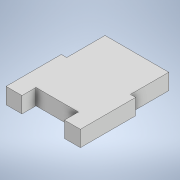
# Autodesk Inventor part: Expansiemodule
Saved by Autodesk Inventor 2021 (Build 250183000, 183)
## iProperties
Created: 2022-02-18
Part Number: Expansiemodule
Material: Generic
Document SubType Name: Modeling
Designer: woutr
Density: 1 g/cm^3
Appearance: Default
Author: woutr
Autodesk Inventor part; units mm, degrees
ref_plane "YZ Plane" through (0, 0, 0) normal (1, 0, 0) x (0, 1, 0)
ref_plane "XZ Plane" through (0, 0, 0) normal (0, 1, 0) x (-1, 0, 0)
ref_plane "XY Plane" through (0, 0, 0) normal (0, 0, 1) x (1, 0, 0)
sketch "Sketch1" plane through (0, 0, 0) normal (0, 1, 0) x (-1, 0, 0)
  line L0 (0, 0) -> (15, 0)
  line L1 (15, 0) -> (15, -13.2)
  line L2 (15, -13.2) -> (55, -13.2)
  line L3 (55, -13.2) -> (55, 0)
  line L4 (55, 0) -> (70, 0)
  line L5 (70, 0) -> (70, -52)
  line L6 (70, -52) -> (64.9, -52)
  line L7 (64.9, -52) -> (64.9, -88.1)
  line L8 (64.9, -88.1) -> (4.9, -88.1)
  line L9 (4.9, -88.1) -> (4.9, -52)
  line L10 (4.9, -52) -> (0, -52)
  line L11 (0, -52) -> (0, 0)
  dimension "d0" = 15
  dimension "d1" = 13.2
  dimension "d2" = 40
  dimension "d3" = 15
  dimension "d4" = 52
  dimension "d5" = 5.1
  dimension "d6" = 36.1
  dimension "d7" = 60
  constraints: 24 end point, 8 perpendicular, 4 point on line, 1 horizontal, 1 vertical
  measures "d0" distance of L0.start L0.end
  measures "d1" distance of L0.end L1.end
  measures "d2" distance of L1.end L2.end
  measures "d3" distance of L3.end L4.end
  measures "d4" distance of L4.end L5.end
  measures "d5" distance of L5.end L6.end
  measures "d6" distance of L6.end L7.end
  measures "d7" distance of L7.end L8.end
extrude "Extrusion1" add sketch "Sketch1" along normal blind 15
body "Solid1"
